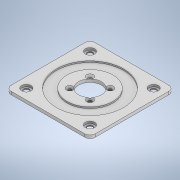
# Autodesk Inventor part: Motor Support Plate
Saved by Autodesk Inventor 2022 (Build 260153000, 153)
## iProperties
Created: 2022-03-02
Part Number: Motor Support Plate
Material: Genérico
Document SubType Name: Modeling
Designer: JK
Density: 1 g/cm^3
Appearance: Valor por defecto
Author: JK
Autodesk Inventor part; units mm, degrees
ref_plane "YZ Plane" through (0, 0, 0) normal (1, 0, 0) x (0, 1, 0)
ref_plane "XZ Plane" through (0, 0, 0) normal (0, 1, 0) x (-1, 0, 0)
ref_plane "XY Plane" through (0, 0, 0) normal (0, 0, 1) x (1, 0, 0)
sketch "Boceto1" plane through (0, 0, 0) normal (0, 1, 0) x (-1, 0, 0)
  circle A0 centre (0, 0) radius 35
  dimension "d0" = 70
  constraints: 1 centre point
  measures "d0" diameter of A0
extrude "Extrusión1" add sketch "Boceto1" along normal blind 3
sketch "Boceto2" plane through (0, 3, 0) normal (0, 1, 0) x (1, 0, 0)
  circle A0 centre (0, 0) radius 22.45
  circle A1 centre (0, 0) radius 32.9
  dimension "d4" = 44.9
  dimension "d5" = 65.8
  constraints: 2 centre point, 2 coincident
  measures "d4" diameter of A0
  measures "d5" diameter of A1
extrude "Extrusión2" cut sketch "Boceto2" against normal blind 1.4
sketch "Boceto3" plane through (0, 3, 0) normal (0, 1, 0) x (1, 0, 0)
  circle A0 centre (0, 0) radius 17.5
  dimension "d8" = 35
  constraints: 1 centre point, 1 coincident
  measures "d8" diameter of A0
extrude "Extrusión3" cut sketch "Boceto3" against normal through all
sketch "Boceto4" plane through (0, 3, 0) normal (0, 1, 0) x (1, 0, 0)
  circle A0 centre (0, 0) radius 17.5 projected
  circle A1 centre (0, 0) radius 11.2
  line L0 (41.2, -41.2) -> (-41.2, -41.2)
  line L1 (-41.2, -41.2) -> (-41.2, 41.2)
  line L2 (-41.2, 41.2) -> (41.2, 41.2)
  line L3 (41.2, 41.2) -> (41.2, -41.2)
  line L4 (41.2, -41.2) -> (-41.2, 41.2) construction
  line L5 (-41.2, -41.2) -> (41.2, 41.2) construction
  circle A2 centre (0, 0) radius 35 projected
  dimension "d11" = 22.4
  dimension "d12" = 82.4
  dimension "d13" = 82.4
  constraints: 12 end point, 2 midpoint, 2 parallel, 1 centre point, 1 coincident, 1 horizontal, 1 perpendicular
  measures "d11" diameter of A1
  measures "d12" distance between parallel lines of L3 L1
  measures "d13" distance of L0.end L1.end
extrude "Extrusión4" add sketch "Boceto4" against normal up to surface (3 mm away)
sketch "Boceto5" plane through (0, 3, 0) normal (0, 1, 0) x (1, 0, 0)
  circle A0 centre (0, 0) radius 14
  circle A1 centre (-9.8995, -9.8995) radius 1.7
  line L0 (0, 0) -> (0, -14)
  line L1 (0, 0) -> (-9.8995, -9.8995)
  circle A2 centre (-31.2, -31.2) radius 2.7
  line L2 (-41.2, 41.2) -> (-41.2, -41.2) projected
  line L3 (-41.2, -41.2) -> (41.2, -41.2) projected
  dimension "d16" = 3.4
  dimension "d17" = 28
  dimension "d18" = 45
  dimension "d21" = 10
  dimension "d22" = 10
  dimension "d23" = 5.4
  constraints: 4 end point, 3 centre point, 2 point on circle, 1 coincident, 1 vertical
  measures "d16" diameter of A1
  measures "d17" diameter of A0
  measures "d18" angle of L1 L0
  measures "d21" distance from line of L2 A2.centre
  measures "d22" distance from line of L3 A2.centre
  measures "d23" diameter of A2
extrude "Extrusión5" cut sketch "Boceto5" against normal through all contours A1 A0 | A0 L1 A1 | A1 L1 A0 | A2
sketch "Boceto6" plane through (0, 3, 0) normal (0, 1, 0) x (1, 0, 0)
  circle A0 centre (-31.2, -31.2) radius 2.7 projected
  circle A1 centre (-31.2, -31.2) radius 4.6
  point P0 (0, 0)
  dimension "d24" = 9.2
  constraints: 1 centre point, 1 coincident
  measures "d24" diameter of A1
extrude "Extrusión6" cut sketch "Boceto6" against normal blind 2
chamfer "Chaflán1" distance 1.6 angle 45 1 edges at (-11.5995, 3, 9.8995)
pattern_circular "Patrón circular1" count 4 over 360 about axis through (0, 3, 0) along (0, -1, 0) of "Extrusión5", "Extrusión6", "Chaflán1"
fillet "Empalme1" radius 5 4 edges at (-41.2, 1.5, 41.2) (41.2, 1.5, 41.2) (41.2, 1.5, -41.2) (-41.2, 1.5, -41.2)
